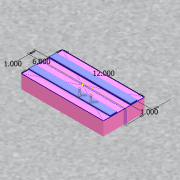
# Autodesk Inventor part: Coupler-3D
Saved by Autodesk Inventor 2017 (Build 210142000, 142)
## iProperties
Created: 2017-07-31
Part Number: Coupler-3D
Material: Generic
Document SubType Name: Modeling
Designer: momar
Density: 1 g/cm^3
Appearance: Default
Author: momar
Autodesk Inventor part; units mm, degrees
ref_plane "YZ Plane" through (0, 0, 0) normal (1, 0, 0) x (0, 1, 0)
ref_plane "XZ Plane" through (0, 0, 0) normal (0, 1, 0) x (-1, 0, 0)
ref_plane "XY Plane" through (0, 0, 0) normal (0, 0, 1) x (1, 0, 0)
sketch "Substrate and Ribbon" plane through (0, 0, 0) normal (0, 1, 0) x (-1, 0, 0)
  line L0 (-152.4, 76.2) -> (152.4, 76.2)
  line L1 (152.4, 76.2) -> (152.4, -76.2)
  line L2 (152.4, -76.2) -> (-152.4, -76.2)
  line L3 (-152.4, -76.2) -> (-152.4, 76.2)
  line L4 (-152.4, 76.2) -> (152.4, -76.2) construction
  line L5 (152.4, 76.2) -> (-152.4, -76.2) construction
  line L6 (152.4, -25.4) -> (-152.4, -25.4)
  line L7 (-152.4, -25.4) -> (-152.4, -50.8)
  line L8 (-152.4, -50.8) -> (152.4, -50.8)
  line L9 (152.4, -50.8) -> (152.4, -25.4)
  line L10 (152.4, 0) -> (-152.4, 0) construction
  point P0 (0, 0)
  dimension "d0" = 304.8
  dimension "d1" = 152.4
  dimension "d2" = 25.4
  dimension "d10" = 25.4
  constraints: 22 end point, 4 midpoint, 4 parallel, 2 horizontal, 2 perpendicular, 2 point on line
  measures "d0" distance of L1.end L2.end
  measures "d1" distance of L0.end L1.end
  measures "d2" distance of L7.end L6.end
  measures "d10" distance between parallel lines of L6 L10
extrude "Graphene Ribbon" add sketch "Substrate and Ribbon" along normal blind 5.08 contours L6 L1 L8 L3
extrude "Substrate" add sketch "Substrate and Ribbon" against normal blind 50.8 separate body
ref_plane "Mirror Plane" through (-152.4, 0, 0) normal (0, 0, -1) x (1, 0, 0)
mirror "Coupled Ribbon" about plane through (-152.4, 0, 0) normal (0, 0, -1) of "Graphene Ribbon" bodies 1
body "Solid1"
body "Solid2"
